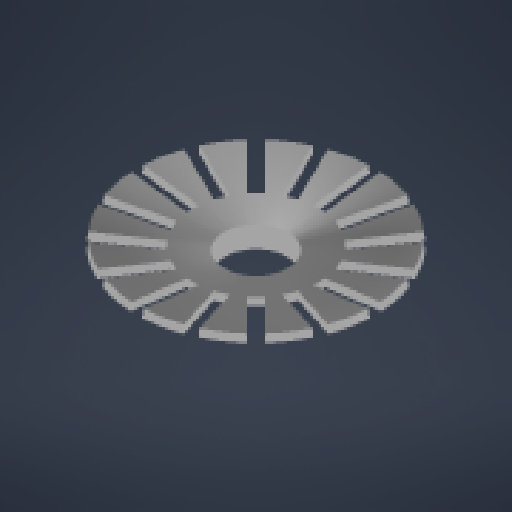
# Autodesk Inventor part: Parte de arriba aspresor
Saved by Autodesk Inventor 2024 (Build 280153000, 153)
## iProperties
Created: 2023-06-25
Part Number: Parte de arriba aspresor
Material: Generic
Document SubType Name: Modeling
Designer: TES
Density: 1 g/cm^3
Appearance: Chrome - Polished
Author: TES
Autodesk Inventor part; units mm, degrees
ref_plane "YZ Plane" through (0, 0, 0) normal (1, 0, 0) x (0, 1, 0)
ref_plane "XY Plane" through (0, 0, 0) normal (0, 0, 1) x (1, 0, 0)
sketch "Sketch1" plane through (0, 0, 0) normal (0, 0, 1) x (1, 0, 0)
  line L0 (0, 0) -> (0, 12.8972) construction
  line L1 (-15, 2) -> (0, 0)
  line L2 (-15.1322, 1.0088) -> (1, -1.1422)
  line L3 (1, -1.1422) -> (1, 12.8972)
  line L4 (-2.5, 0.3333) -> (-2.5, -0.6755)
  line L5 (-15, 2) -> (-15.1322, 1.0088)
  dimension "d2" = 1
  dimension "d3" = 2.5
  constraints: 12 end point, 2 point on line, 2 vertical, 1 other
  measures "d2" distance between parallel lines of L1 L2
  measures "d3" distance between parallel lines of L0 L4
revolve "Revolution1" add sketch "Sketch1" angle 360 about axis through (0, 0, 0) along (0, 1, 0)
ref_plane "Work Plane1" through (0, 4, 0) normal (0, 1, 0) x (-1, 0, 0)
sketch "Sketch2" plane through (0, 4, 0) normal (0, 1, 0) x (-1, 0, 0)
  circle A0 centre (0, 0) radius 15.1322
  circle A1 centre (0, 0) radius 15.1322 projected
  circle A2 centre (0, 0) radius 8
  line L0 (0, -8) -> (0, -15.8573) construction
  line L1 (-0.75, -7.9648) -> (-0.75, -15.8573)
  line L2 (0.75, -7.9648) -> (0.75, -15.8573)
  point P0 (0.75, -15.1136)
  point P1 (-0.75, -15.1136)
  dimension "d6" = 16
  dimension "d7" = 0.75
  dimension "d8" = 0.75
  constraints: 6 end point, 3 point on circle, 2 centre point, 2 coincident, 2 parallel, 1 vertical
  measures "d6" diameter of A2
  measures "d7" distance between parallel lines of L0 L1
  measures "d8" distance between parallel lines of L0 L2
extrude "Extrusion1" cut sketch "Sketch2" against normal blind 10 contours L1 A2 L2 A0 picked at (0.5834, -10.3582)
pattern_circular "Circular Pattern1" count 16 over 360 about axis through (0, 1.1667, 0) along (0, 1, 0) of "Extrusion1"
ref_plane "Work Plane2" through (0, -0.7, 0) normal (0, 1, 0) x (-1, 0, 0)
sketch "Sketch3" plane through (0, -0.7, 0) normal (0, 1, 0) x (-1, 0, 0)
  circle A0 centre (0, 0) radius 4
  circle A1 centre (0, 0) radius 2.5 projected
  dimension "d15" = 8
  constraints: 1 centre point, 1 coincident
  measures "d15" diameter of A0
extrude "Extrusion2" add sketch "Sketch3" along normal blind 1.5
fillet "Fillet1" radius 0.5 2 edges at (4, 0.8, 0) (2.5, 0.8, 0)
sketch "Sketch4" plane through (0, -0.7, 0) normal (0, 1, 0) x (-1, 0, 0)
  circle A0 centre (0, 0) radius 4
  dimension "d19" = 8
  constraints: 1 centre point, 1 coincident
  measures "d19" diameter of A0
extrude "Extrusion3" add sketch "Sketch4" against normal blind 4
fillet "Fillet6" radius 2 1 edges at (4, -0.4755, 0)
sketch "Boceto21" plane through (0, -4.7, 0) normal (0, -1, 0) x (1, 0, 0)
  circle A0 centre (0, 0) radius 4
  constraints: 1 centre point, 1 coincident
extrude "Extrusión19" cut sketch "Boceto21" against normal blind 100
scale "Escala1" factors (4, 4, 4) then translate (0, -3.8, 0) bodies 1
body "Solid1"
